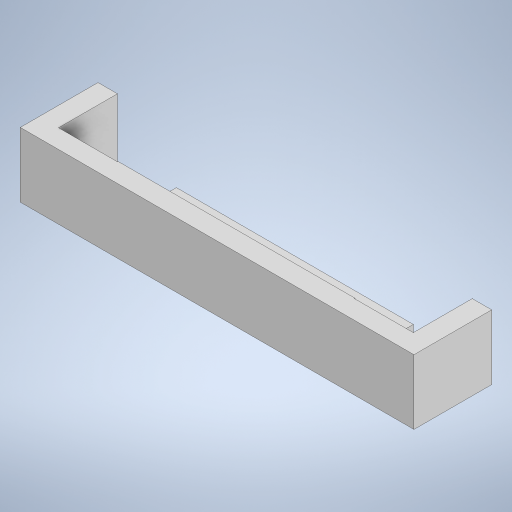
# Autodesk Inventor part: VerticalAxis
Saved by Autodesk Inventor 2024 (Build 280153000, 153)
## iProperties
Created: 2023-11-28
Part Number: VerticalAxis
Material: Generic
Document SubType Name: Modeling
Designer: KirikDK
Density: 1 g/cm^3
Appearance: Default
Author: KirikDK
Autodesk Inventor part; units mm, degrees
ref_plane "YZ Plane" through (0, 0, 0) normal (1, 0, 0) x (0, 1, 0)
ref_plane "XZ Plane" through (0, 0, 0) normal (0, 1, 0) x (-1, 0, 0)
ref_plane "XY Plane" through (0, 0, 0) normal (0, 0, 1) x (1, 0, 0)
sketch "Sketch1" plane through (0, 0, 0) normal (0, 1, 0) x (-1, 0, 0)
  line L0 (119.875, 68.5) -> (-154.125, 68.5)
  line L1 (-154.125, 68.5) -> (-154.125, 8.5)
  line L2 (-154.125, 8.5) -> (119.875, 8.5)
  line L3 (119.875, 8.5) -> (119.875, 68.5)
  point P0 (0, 0)
  dimension "d0" = 274
  dimension "d1" = 60
  constraints: 8 end point, 2 parallel, 1 horizontal, 1 perpendicular
  measures "d0" distance of L0.start L0.end
  measures "d1" distance of L2.end L0.start
extrude "Extrusion1" add sketch "Sketch1" along normal blind 10
sketch "Sketch2" plane through (0, 10, 0) normal (0, 1, 0) x (1, 0, 0)
  line L0 (-119.875, -8.5) -> (-119.875, -68.5) projected
  line L1 (-119.875, -68.5) -> (154.125, -68.5)
  line L2 (154.125, -68.5) -> (154.125, -53.5)
  line L3 (154.125, -53.5) -> (-119.875, -53.5)
  line L4 (-119.875, -53.5) -> (-119.875, -68.5)
  line L5 (154.125, -68.5) -> (154.125, -8.5) projected
  line L6 (154.125, -8.5) -> (-119.875, -8.5) projected
  line L7 (-119.875, -8.5) -> (-119.875, -68.5) projected
  line L8 (-119.875, -68.5) -> (154.125, -68.5) projected
  point P0 (0, 0)
  dimension "d4" = 15
  constraints: 8 end point, 2 parallel, 1 horizontal, 1 perpendicular
  measures "d4" distance of L1.end L2.end
extrude "Extrusion2" add sketch "Sketch2" along normal blind 50 contours L3 L2 L1 L0
sketch "Sketch3" plane through (0, 10, 0) normal (0, 1, 0) x (1, 0, 0)
  line L0 (154.125, -8.5) -> (108.625, -8.5)
  line L1 (108.625, -8.5) -> (108.625, -54)
  line L2 (108.625, -54) -> (154.125, -54)
  line L3 (154.125, -54) -> (154.125, -8.5)
  line L4 (-119.875, -8.5) -> (-119.875, -68.5) projected
  line L5 (-119.875, -8.5) -> (-74.375, -8.5)
  line L6 (-74.375, -8.5) -> (-74.375, -54)
  line L7 (-74.375, -54) -> (-119.875, -54)
  line L8 (-119.875, -54) -> (-119.875, -8.5)
  point P0 (0, 0)
  dimension "d7" = 45.5
  dimension "d8" = 45.5
  constraints: 16 end point, 4 parallel, 2 horizontal, 2 perpendicular
  measures "d7" distance of L0.start L0.end
  measures "d8" distance of L4.start L5.end
extrude "Extrusion3" cut sketch "Sketch3" along normal mid plane 150
sketch "Sketch4" plane through (0, 0, 0) normal (0, -1, 0) x (1, 0, 0)
  line L0 (-74.375, 54) -> (-74.375, 8.5) projected
  line L1 (108.625, 8.5) -> (-74.375, 8.5) projected
  line L2 (108.625, 8.5) -> (108.625, 54) projected
  line L3 (108.625, 54) -> (154.125, 54) projected
  line L4 (154.125, 68.5) -> (154.125, 54) projected
  line L5 (-119.875, 68.5) -> (154.125, 68.5) projected
  line L6 (-119.875, 54) -> (-119.875, 68.5) projected
  line L7 (-119.875, 54) -> (-74.375, 54) projected
  line L8 (-119.875, 68.5) -> (-134.875, 68.5)
  line L9 (-134.875, 68.5) -> (-134.875, 8.5)
  line L10 (-134.875, 8.5) -> (-119.875, 8.5)
  line L11 (-119.875, 8.5) -> (-119.875, 68.5)
  line L12 (154.125, 68.5) -> (169.125, 68.5)
  line L13 (169.125, 68.5) -> (169.125, 8.5)
  line L14 (169.125, 8.5) -> (154.125, 8.5)
  line L15 (154.125, 8.5) -> (154.125, 68.5)
  point P0 (0, 0)
  dimension "d11" = 60
  dimension "d12" = 60
  dimension "d13" = 15
  dimension "d14" = 15
  constraints: 16 end point, 4 parallel, 2 horizontal, 2 perpendicular
  measures "d11" distance of L8.end L9.end
  measures "d12" distance of L12.end L13.end
  measures "d13" distance of L13.end L14.end
  measures "d14" distance of L9.end L10.end
extrude "Extrusion4" add sketch "Sketch4" against normal blind 50 contours L11 L10 L9 L8 L6 | L12 L13 L14 L15 L4
sketch "Sketch5" plane through (0, 60, 0) normal (0, 1, 0) x (1, 0, 0)
  line L0 (-140, -80) -> (185, -80)
  line L1 (185, -80) -> (185, 19)
  line L2 (185, 19) -> (-140, 19)
  line L3 (-140, 19) -> (-140, -80)
  point P0 (0, 0)
  constraints: 8 end point, 2 parallel, 1 horizontal, 1 perpendicular
extrude "Extrusion5" cut sketch "Sketch5" against normal up to surface (10 mm away)
body "Solid1"
